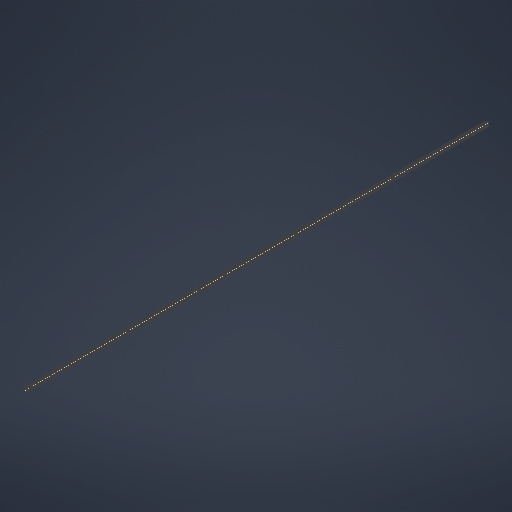
# Autodesk Inventor part: SP40-01 MARCO BATIENTE - PAÑO
Saved by Autodesk Inventor 2025 (Build 290162000, 162)
## iProperties
Created: 2026-01-17
Part Number: SP40-01 MARCO BATIENTE - PAÑO
Material: Aluminio
Document SubType Name: Modeling
Designer: ROLANDO
Density: 2.7 g/cm^3
Appearance: Satinado
Author: ROLANDO
Autodesk Inventor part; units mm, degrees
ref_plane "YZ Plane" through (0, 0, 0) normal (1, 0, 0) x (0, 1, 0)
ref_plane "XZ Plane" through (0, 0, 0) normal (0, 1, 0) x (-1, 0, 0)
ref_plane "XY Plane" through (0, 0, 0) normal (0, 0, 1) x (1, 0, 0)
sketch "Boceto1" plane through (0, 0, 0) normal (0, 0, 1) x (1, 0, 0)
  line L0 (-31.2865, 21.2119) -> (-31.2865, 0.1784)
  line L1 (-29.3865, 4.1784) -> (11.8135, 4.1784)
  line L2 (13.7135, 0.1784) -> (13.7135, 15.8119)
  line L3 (9.0135, 44.1784) -> (9.0135, 21.5886)
  line L4 (9.0135, 44.1784) -> (3.8135, 44.1784)
  line L5 (5.2135, 42.7784) -> (7.6135, 42.7784)
  line L6 (7.6135, 36.2784) -> (5.2135, 36.2784)
  line L7 (-29.8865, 19.8119) -> (8.3135, 19.8119)
  line L8 (12.3135, 15.8119) -> (12.3135, 6.0784)
  line L9 (11.8135, 5.5784) -> (-29.3865, 5.5784)
  line L10 (-29.8865, 6.0784) -> (-29.8865, 19.8119)
  arc A0 (13.7135, 15.8119) -> (9.4118, 21.099) centre (8.3135, 15.8119) ccw
  arc A1 (12.3135, 15.8119) -> (8.3135, 19.8119) centre (8.3135, 15.8119) ccw
  line L11 (12.3135, 3.6784) -> (12.3135, 1.9253)
  line L12 (11.2135, 0.1784) -> (13.7135, 0.1784)
  line L13 (7.6135, 21.6784) -> (7.6135, 34.8784)
  line L14 (7.6135, 36.2784) -> (7.6135, 42.7784)
  line L15 (-29.8865, 3.6784) -> (-29.8865, 1.8562)
  line L16 (-28.7865, 0.1784) -> (-31.2865, 0.1784)
  line L17 (-28.7865, 0.1784) -> (-28.7865, 0.6338)
  line L18 (11.2135, 0.1784) -> (11.2135, 0.8784)
  line L19 (-29.8865, 21.1784) -> (-29.8865, 24.1784)
  line L20 (-28.7665, 25.5784) -> (-31.2865, 25.5784)
  line L21 (-31.2865, 25.5784) -> (-31.2865, 21.2119)
  line L22 (-10.2865, 21.1784) -> (-10.2865, 25.5784)
  line L23 (-10.2865, 25.5784) -> (-12.6765, 25.5784)
  line L24 (-11.6865, 24.1784) -> (-11.6865, 21.1784)
  line L25 (7.1135, 21.1784) -> (-10.2865, 21.1784)
  line L26 (-11.6865, 21.1784) -> (-29.8865, 21.1784)
  line L27 (-27.8865, 24.1784) -> (-29.8865, 24.1784)
  line L28 (-13.6865, 24.1784) -> (-11.6865, 24.1784)
  line L29 (-29.0312, 1.0637) -> (-29.6418, 1.4262)
  line L30 (11.2135, 0.8784) -> (12.1053, 1.5192)
  line L31 (-27.8865, 24.1784) -> (-27.8865, 24.8734)
  line L32 (-13.6865, 24.1784) -> (-13.6865, 24.8843)
  line L33 (-28.7665, 25.5784) -> (-27.8865, 24.8734)
  line L34 (-13.6865, 24.8843) -> (-12.6765, 25.5784)
  line L35 (7.6135, 34.8784) -> (3.8135, 34.8784)
  line L36 (5.2135, 37.5284) -> (5.2135, 36.2784)
  line L37 (5.2135, 41.5284) -> (5.2135, 42.7784)
  line L38 (5.2135, 37.5284) -> (4.5077, 37.5284)
  line L39 (5.2135, 41.5284) -> (4.5077, 41.5284)
  line L40 (3.8135, 44.1784) -> (3.8135, 42.5384)
  line L41 (3.8135, 42.5384) -> (4.5077, 41.5284)
  line L42 (3.8135, 34.8784) -> (3.8135, 36.5184)
  line L43 (3.8135, 36.5184) -> (4.5077, 37.5284)
  arc A2 (7.1135, 21.1784) -> (7.6135, 21.6784) centre (7.1135, 21.6784) ccw
  arc A3 (9.0135, 21.5886) -> (9.4118, 21.099) centre (9.5135, 21.5886) ccw
  arc A4 (11.8135, 5.5784) -> (12.3135, 6.0784) centre (11.8135, 6.0784) ccw
  arc A5 (12.3135, 3.6784) -> (11.8135, 4.1784) centre (11.8135, 3.6784) ccw
  arc A6 (12.1053, 1.5192) -> (12.3135, 1.9253) centre (11.8135, 1.9253) ccw
  arc A7 (-29.8865, 6.0784) -> (-29.3865, 5.5784) centre (-29.3865, 6.0784) ccw
  arc A8 (-29.3865, 4.1784) -> (-29.8865, 3.6784) centre (-29.3865, 3.6784) ccw
  arc A9 (-29.8865, 1.8562) -> (-29.6418, 1.4262) centre (-29.3865, 1.8562) ccw
  line L44 (13.7135, 4.1784) -> (13.7135, 4.2119)
  arc A10 (-28.7865, 0.6338) -> (-29.0312, 1.0637) centre (-29.2865, 0.6338) ccw
  point P0 (0, 0)
  point P1 (5.2135, 42.1534)
  point P2 (-28.7865, 4.1784)
  point P3 (7.6135, 39.5284)
  point P4 (-28.7865, 0.9184)
  dimension "d16" = 5.4
  dimension "d17" = 4
  dimension "d32" = 1.4
  dimension "d35" = 1.4
  dimension "d37" = 3
  dimension "d38" = 25.4
  dimension "d44" = 18.2
  dimension "d50" = 0.7
  dimension "d53" = 40.3
  dimension "d54" = 37.5
  dimension "d55" = 1.4
  dimension "d57" = 17
  dimension "d62" = 30.7
  dimension "d63" = 35.7
  dimension "d64" = 4.4
  dimension "d66" = 3
  dimension "d69" = 4.4
  dimension "d71" = 3.4
  dimension "d72" = 3.4
  dimension "d73" = 0.88
  dimension "d74" = 1.01
  dimension "d75" = 34.5
  dimension "d76" = 38.7
  dimension "d77" = 0.695
  dimension "d78" = 0.7058
  dimension "d81" = 23
  dimension "d82" = 44
  dimension "d84" = 6.5
  dimension "d85" = 2.4
  dimension "d86" = 2.4
  dimension "d87" = 9.3
  dimension "d88" = 1.4
  dimension "d99" = 1.4
  dimension "d100" = 1.4
  dimension "d102" = 1.4
  dimension "d140" = 111
  dimension "d141" = 4
  dimension "d142" = 6.02
  dimension "d143" = 0.7058
  dimension "d144" = 0.7058
  dimension "d199" = 1.4
  dimension "d201" = 14.2
  dimension "d202" = 0.5
  dimension "d203" = 3.01
  dimension "d204" = 2
  dimension "d205" = 2.5
  dimension "d206" = 4.7
  dimension "d207" = 6.1
  dimension "d208" = 42.5
  dimension "d209" = 41.35
  dimension "d210" = 5.4
  dimension "d211" = 4
  dimension "d212" = 19.6335
  dimension "d213" = 13.7135
  dimension "d216" = 4.0335
  dimension "d218" = 0.74
  dimension "d219" = 0.5
  dimension "d220" = 45
  dimension "d221" = 5.2
  constraints: 90 end point, 22 point on circle, 21 tangent, 13 parallel, 11 centre point, 9 horizontal, 7 equal radius, 6 perpendicular, 5 collinear, 5 point on line, 4 vertical, 2 midpoint, 1 coincident, 1 equal length
  measures "d16" radius of A0
  measures "d17" radius of A1
  measures "d32" distance between parallel lines of L22 L24
  measures "d35" distance between parallel lines of L19 L21
  measures "d37" distance between parallel lines of L26 L28
  measures "d38" distance between parallel lines of L16 L20
  measures "d44" distance between parallel lines of L24 L19
  measures "d50" distance of L12.start L18.end
  measures "d53" distance between parallel lines of L0 L3
  measures "d54" distance between parallel lines of L10 L14
  measures "d55" distance between parallel lines of L3 L14
  measures "d57" distance between parallel lines of L1 L26
  measures "d62" angle of L16 L29
  measures "d63" angle of L12 L30
  measures "d64" distance between parallel lines of L20 L26
  measures "d66" distance between parallel lines of L26 L27
  measures "d69" distance between parallel lines of L26 L23
  measures "d71" distance between parallel lines of L22 L32
  measures "d72" distance between parallel lines of L21 L31
  measures "d73" distance from line of L31 L20.start
  measures "d74" distance from line of L32 L23.end
  measures "d75" angle of L23 L34
  measures "d76" angle of L20 L33
  measures "d77" distance of L27.start L31.end
  measures "d78" distance of L28.start L32.end
  measures "d81" distance between parallel lines of L25 L4
  measures "d82" distance between parallel lines of L12 L4
  measures "d84" distance between parallel lines of L6 L5
  measures "d85" distance from line of L5.start L14
  measures "d86" distance of L6.start L6.end
  measures "d87" distance between parallel lines of L35 L4
  measures "d88" distance between parallel lines of L35 L6
  measures "d99" distance between parallel lines of L4 L5
  measures "d100" distance from line of point (5.214, 42.153) L40
  measures "d102" distance between parallel lines of L36 L42
  measures "d140" angle of L43 L41
  measures "d141" distance between parallel lines of L38 L39
  measures "d142" distance of L42.end L40.end
  measures "d143" distance of L37.start L39.end
  measures "d144" distance of L36.start L38.end
  measures "d199" radial gap between concentric circles of A0 A1
  measures "d201" distance between parallel lines of L32 L31
  measures "d202" radius of A2
  measures "d203" vertical distance of point (7.614, 39.528) L40.end
  measures "d204" distance from line of point (7.614, 39.528) L39
  measures "d205" distance between parallel lines of L2 L18
  measures "d206" distance between parallel lines of L2 L3
  measures "d207" distance between parallel lines of L2 L14
  measures "d208" distance between parallel lines of L2 L17
  measures "d209" distance between parallel lines of L12 L39
  measures "d210" distance between parallel lines of L9 L12
  measures "d211" distance between parallel lines of L1 L12
  measures "d212" distance between parallel lines of L7 L12
  measures "d213" distance from line of point (0, 0) L2
  measures "d216" distance from line of L44.end L12
  measures "d218" distance of L16.start point (-28.786, 0.918)
  measures "d219" radius of A10
  measures "d220" distance between parallel lines of L2 L0
  measures "d221" distance between parallel lines of L40 L3
extrude "Extrusión1" add sketch "Boceto1" against normal blind 5000
